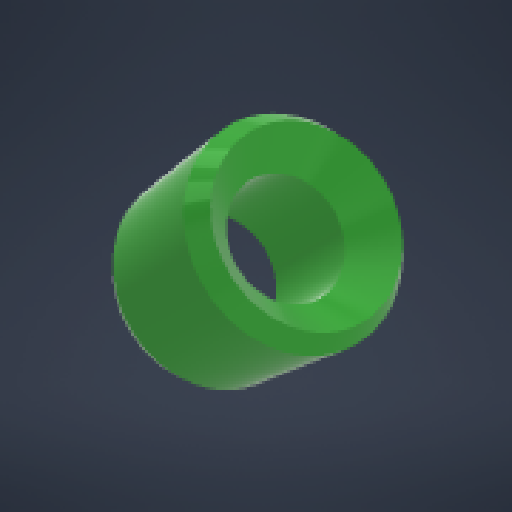
# Autodesk Inventor part: Roller
Saved by Autodesk Inventor 2023.1 (Build 271208000, 208)
## iProperties
Created: 2022-11-26
Part Number: Roller
Material: PC/ABS Plastic
Document SubType Name: Modeling
Designer: aubrey-work
Density: 0.357273 g/cm^3
Appearance: Smooth - Dark Forest Green
Author: aubrey-work
Autodesk Inventor part; units mm, degrees
ref_plane "YZ Plane" through (0, 0, 0) normal (1, 0, 0) x (0, 1, 0)
ref_plane "XZ Plane" through (0, 0, 0) normal (0, 1, 0) x (-1, 0, 0)
ref_plane "XY Plane" through (0, 0, 0) normal (0, 0, 1) x (1, 0, 0)
derived "Slew Bearing Master.ipt"
sketch "Sketch1" plane through (0, 0, 0) normal (0, 1, 0) x (-1, 0, 0)
  circle A0 centre (0, 0) radius 51.7779
  ellipse E0 centre (-51.7779, 0) end of major axis (-57.5055, 0) minor radius 4.05
  line L0 (-46.0503, 0) -> (-57.5055, 0)
  line L1 (-51.7779, -4.05) -> (-51.7779, 4.05)
  line L2 (0, 0) -> (-51.7779, 0)
  line L3 (0, 0) -> (-51.1443, -4.0251)
sketch "Sketch2" plane through (0, 0, 0) normal (0, 0, 1) x (1, 0, 0)
  line L0 (57.5055, 0) -> (46.0503, 0)
  line L1 (46.0503, 0) -> (51.7779, -5.7276)
  line L2 (51.7779, -5.7276) -> (57.5055, 0)
  line L3 (57.5055, 0) -> (51.7779, 5.7276)
  line L4 (51.7779, 5.7276) -> (46.0503, 0)
  line L5 (48.9141, 2.8638) -> (54.6417, -2.8638)
  line L6 (48.9141, -2.8638) -> (54.6417, 2.8638)
  line L7 (51.7779, 5.7276) -> (51.7779, -5.7276)
  line L8 (57.162, 0) -> (61.762, 0)
  line L9 (61.762, 0) -> (61.762, -5.7276)
  line L10 (61.762, -5.7276) -> (52.5779, -5.7276)
  line L11 (52.5779, -5.7276) -> (52.5779, -4.9983)
  line L12 (52.5779, -4.9983) -> (56.8691, -0.7071)
  arc A0 (56.8691, -0.7071) -> (57.162, 0) centre (56.162, 0) ccw
  arc A1 (57.162, 0) -> (56.8691, 0.7071) centre (56.162, 0) ccw
  line L13 (52.5779, 4.9983) -> (56.8691, 0.7071)
  line L14 (52.5779, 5.7276) -> (52.5779, 4.9983)
  line L15 (61.762, 5.7276) -> (52.5779, 5.7276)
  line L16 (61.762, 0) -> (61.762, 5.7276)
  line L17 (50.9779, 5.7276) -> (50.9779, 4.9983)
  line L18 (41.7938, 5.7276) -> (50.9779, 5.7276)
  line L19 (50.9779, 4.9983) -> (46.6867, 0.7071)
  line L20 (41.7938, 0) -> (41.7938, 5.7276)
  line L21 (41.7938, 0) -> (41.7938, -5.7276)
  arc A2 (46.6867, 0.7071) -> (46.3938, 0) centre (47.3938, 0) ccw
  arc A3 (46.3938, 0) -> (46.6867, -0.7071) centre (47.3938, 0) ccw
  line L22 (50.9779, -4.9983) -> (46.6867, -0.7071)
  line L23 (46.3938, 0) -> (41.7938, 0)
  line L24 (50.9779, -5.7276) -> (50.9779, -4.9983)
  line L25 (41.7938, -5.7276) -> (50.9779, -5.7276)
  line L26 (59.462, 5.7276) -> (59.462, -5.7276)
  line L27 (60.962, 5.7276) -> (60.962, -5.7276)
  line L28 (57.962, 5.7276) -> (57.962, -5.7276)
  line L29 (45.5938, 5.7276) -> (45.5938, -5.7276)
  line L30 (44.0938, 5.7276) -> (44.0938, -5.7276)
  line L31 (55.8891, 1.0506) -> (50.7273, -4.1113)
  line L32 (50.7273, -4.1113) -> (51.2823, -4.6662)
  line L33 (51.2823, -4.6662) -> (52.425, -4.36)
  line L34 (52.425, -4.36) -> (56.4628, -0.972)
  line L35 (56.4628, -0.972) -> (56.769, 0.1708)
  line L36 (56.769, 0.1708) -> (55.8891, 1.0506)
  line L37 (56.4628, -0.972) -> (52.7499, -4.6849)
  line L38 (52.7499, -4.6849) -> (52.425, -4.36)
  point P0 (0, 0)
  point P1 (53.3082, -1.5303)
  point P2 (56.7232, 0)
  point P3 (54.8385, 0)
  point P4 (51.7779, -3.0606)
  point P5 (51.7779, -4.5334)
revolve "Revolution2" add sketch "Sketch2" angle 360 about axis through (48.9141, -2.8638, 0) along (0.7071068, 0.7071068, 0) contours L35 L34 L5 L31 L0 | L5 L34 L33 L7 L31
equation "\"gap\" = 0.1"
equation "\"airgap\" = 0.4"
equation "\"wallgap\" = 0.8"
equation "\"roller_outerDiameter\" = 8"
equation "\"roller_diameter\" = 8"
equation "\"bolt_diameter\" = 3"
equation "\"outerBolt_diameter\" = 3"
equation "\"innerBolt_diameter\" = 3"
equation "\"elephantsFoot\" = 0.4"
